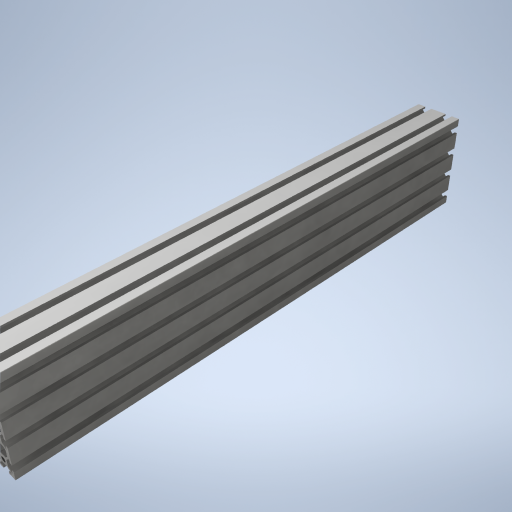
# Autodesk Inventor part: HFSP5-4080-425
Saved by Autodesk Inventor 2024 (Build 280153000, 153)
## iProperties
Category: PARTsolutions
Company: MISUMI
Created: 2024-08-01
Part Number: HFSP5-4080-425
Material: Aluminum 6061
Catalog Web Link: www.cadenas.de
Description: HFSP5-2040, HFSP5-2550, HFSP5-2060, HFSP5-2080, HFSP5-4060, HFSP5-4080-HFS5 Series -Aluminum Extrusion with Milled Surfaces/Rectangle (Vertical)-
Vendor: MISUMI
Document SubType Name: Modeling
Designer: psAdmin
Manufacturer: MISUMI
Mass: 1120.02 g
Surface Area: 3756.67 cm^2
Volume: 414.823 cm^3
Density: 2.7 g/cm^3
Appearance: Anodized - Light Gray
PSOL_IDENT_0: {$CADENAS_DATA/23d-libs/misumi/metric/38_al_extrusions_blackets/5/hfsp5_2040.prj},334 {VTYP=3D},{NB=
PSOL_IDENT_1: HFSP5-4080-425},{LINA=HFSP5-4080-425},{NN=HFSP5-2040, HFSP5-2550, HFSP5-2060, HFSP5-2080, HFSP5-4060
PSOL_IDENT_2: , HFSP5-4080},{DATE=31.05.2023 08:06:28},{GEOMDATE=27.07.2021 03:20:00},{VERSION=},{LINEID=130},{WBV
PSOL_IDENT_3: AR=L,ALT1,ALT10,NH10,AV,BV,CV,DV,EV,ALT12,Z,NH12,XA,XB,XC,XD,XE},{WBNUMERIC=L,NH10,AV,BV,CV,DV,EV,NH
PSOL_IDENT_4: 12,XA,XB,XC,XD,XE}  {NB=HFSP5-4080-425},{LINA=HFSP5-4080-425},{KT=DUMMY},{PN=HFSP5-4080-425},{TPS=HF
PSOL_IDENT_5: SP5-4080},{MAT=A6N01SS-T5  Aluminum Alloy},{ST=Anodize},{FRMH=80},{FRMW=40},{FRD=4.2},{L=425.0},{FS=
PSOL_IDENT_6: HFS5},{T=79.2},{A=40},{ALT1=},{M1=0},{IDM1=4.134},{DALT1=4.2},{DPL1=0},{DPR1=0},{ALT1PN=},{ALT10=},{
PSOL_IDENT_7: ALT10ALG= '','w/o Location Specified Wrench Access Hole Alteratons (Vertical)','1','with Location Sp
PSOL_IDENT_8: ecified Wrench Access Hole Alteratons (Vertical)' },{D6=N/A},{DD6=0},{DD6ALG=0},{DD6PN=},{NH10=0},{N
PSOL_IDENT_9: H10MAX=5},{NH10ALG=[0]},{AV=0.0},{AVMIN=7},{AVMAX=420},{AVALG=[0]},{BV=0.0},{BVMIN=2},{BVMAX=422},{B
PSOL_IDENT_10: VALG=[0]},{CV=0.0},{CVMIN=2},{CVMAX=424},{CVALG=[0]},{DV=0.0},{DVMIN=2},{DVMAX=426},{DVALG=[0]},{EV=
PSOL_IDENT_11: 0.0},{EVMIN=2},{EVMAX=418},{EVALG=[0]},{ALT9PN=},{ALT10PN=},{ALT11PN=},{ALT12=},{ALT12ALG= '','N/A'
PSOL_IDENT_12: },{Z=},{ZALG= '','N/A' },{DD12=0.0},{DD112=0.0},{NH12=0},{NH12MAX=5},{NH12ALG=[0]},{XA=0.0},{XAMIN=7
PSOL_IDENT_13: },{XAMAX=420},{XAALG=[0]},{XB=0.0},{XBMIN=2},{XBMAX=422},{XBALG=[0]},{XC=0.0},{XCMIN=2},{XCMAX=424},
PSOL_IDENT_14: {XCALG=[0]},{XD=0.0},{XDMIN=2},{XDMAX=426},{XDALG=[0]},{XE=0.0},{XEMIN=2},{XEMAX=418},{XEALG=[0]},{A
PSOL_IDENT_15: LT12PN=},{ERRORALT01=OK},{ERRORALT1012=OK},{ERRORPN=}
NB: HFSP5-4080-425
NN: HFSP5-2040, HFSP5-2550, HFSP5-2060, HFSP5-2080, HFSP5-4060, HFSP5-4080
NT: HFS5 Series -Aluminum Extrusion with Milled Surfaces/Rectangle (Vertical)-
NBSYN: $PN.
LINA: HFSP5-4080-425
CATALOG: Misumi
PN: HFSP5-4080-425
TPS: HFSP5-4080
MAT: A6N01SS-T5  Aluminum Alloy
ST: Clear Anodizing
L: 425
FS: HFS5
T: 79.2
A: 40
ALT1: w/o End Tapping
M1: 0
DPL1: 0
DPR1: 0
ALT10: w/o Location Specified Wrench Access Hole Alteratons (Vertical)
D6: N/A
NH10: 0
AV: 0
BV: 0
CV: 0
DV: 0
EV: 0
ALT12: N/A
Z: N/A
DD12: 0
DD112: 0
NH12: 0
XA: 0
XB: 0
XC: 0
XD: 0
XE: 0
SUPPLIER: MISUMI
ARTICLENO: HFSP5-4080-425
BOMINFO: HFSP5-4080-425
CREATOR: CADENAS GmbH
Title: HFSP5-4080-425
Author: Cadenas PARTsolutions
Comments: HFS5 Series -Aluminum Extrusion with Milled Surfaces/Rectangle (Vertical)-
Autodesk Inventor part; units mm, degrees
ref_plane "YZ Plane" through (0, 0, 0) normal (1, 0, 0) x (0, 1, 0)
ref_plane "XZ Plane" through (0, 0, 0) normal (0, 1, 0) x (-1, 0, 0)
ref_plane "XY Plane" through (0, 0, 0) normal (0, 0, 1) x (1, 0, 0)
sketch "Sketch_118" plane through (0, 0, 0) normal (0, 0, 1) x (1, 0, 0)
  line L0 (-20, -27) -> (-18, -27)
  line L1 (-18, -27) -> (-18, -24)
  line L2 (-18, -24) -> (-17.0607, -24)
  line L3 (-17.0607, -24) -> (-14, -27.0607)
  line L4 (-14, -27.0607) -> (-14, -29.4804)
  line L5 (-14, -29.4804) -> (-13.7, -30)
  line L6 (-13.7, -30) -> (-14, -30.5196)
  line L7 (-14, -30.5196) -> (-14, -32.9393)
  line L8 (-14, -32.9393) -> (-17.0607, -36)
  line L9 (-17.0607, -36) -> (-18, -36)
  line L10 (-18, -36) -> (-18, -33)
  line L11 (-18, -33) -> (-20, -33)
  line L12 (-20, -33) -> (-20, -39)
  arc A0 (-20, -39) -> (-19.8, -39.6) centre (-19, -39) ccw
  line L13 (-19.8, -39.6) -> (-13, -39.6)
  line L14 (-13, -39.6) -> (-13, -38)
  line L15 (-13, -38) -> (-16, -38)
  line L16 (-16, -38) -> (-16, -37.0607)
  line L17 (-16, -37.0607) -> (-12.9393, -34)
  line L18 (-12.9393, -34) -> (-10.5196, -34)
  line L19 (-10.5196, -34) -> (-10, -33.7)
  line L20 (-10, -33.7) -> (-9.4804, -34)
  line L21 (-9.4804, -34) -> (-7.0607, -34)
  line L22 (-7.0607, -34) -> (-4, -37.0607)
  line L23 (-4, -37.0607) -> (-4, -38)
  line L24 (-4, -38) -> (-7, -38)
  line L25 (-7, -38) -> (-7, -39.6)
  line L26 (-7, -39.6) -> (7, -39.6)
  line L27 (7, -39.6) -> (7, -38)
  line L28 (7, -38) -> (4, -38)
  line L29 (4, -38) -> (4, -37.0607)
  line L30 (4, -37.0607) -> (7.0607, -34)
  line L31 (7.0607, -34) -> (9.4804, -34)
  line L32 (9.4804, -34) -> (10, -33.7)
  line L33 (10, -33.7) -> (10.5196, -34)
  line L34 (10.5196, -34) -> (12.9393, -34)
  line L35 (12.9393, -34) -> (16, -37.0607)
  line L36 (16, -37.0607) -> (16, -38)
  line L37 (16, -38) -> (13, -38)
  line L38 (13, -38) -> (13, -39.6)
  line L39 (13, -39.6) -> (19.8, -39.6)
  arc A1 (19.8, -39.6) -> (20, -39) centre (19, -39) ccw
  line L40 (20, -39) -> (20, -33)
  line L41 (20, -33) -> (18, -33)
  line L42 (18, -33) -> (18, -36)
  line L43 (18, -36) -> (17.0607, -36)
  line L44 (17.0607, -36) -> (14, -32.9393)
  line L45 (14, -32.9393) -> (14, -30.5196)
  line L46 (14, -30.5196) -> (13.7, -30)
  line L47 (13.7, -30) -> (14, -29.4804)
  line L48 (14, -29.4804) -> (14, -27.0607)
  line L49 (14, -27.0607) -> (17.0607, -24)
  line L50 (17.0607, -24) -> (18, -24)
  line L51 (18, -24) -> (18, -27)
  line L52 (18, -27) -> (20, -27)
  line L53 (20, -27) -> (20, -13)
  line L54 (20, -13) -> (18, -13)
  line L55 (18, -13) -> (18, -16)
  line L56 (18, -16) -> (17.0607, -16)
  line L57 (17.0607, -16) -> (14, -12.9393)
  line L58 (14, -12.9393) -> (14, -10.5196)
  line L59 (14, -10.5196) -> (13.7, -10)
  line L60 (13.7, -10) -> (14, -9.4804)
  line L61 (14, -9.4804) -> (14, -7.0607)
  line L62 (14, -7.0607) -> (17.0607, -4)
  line L63 (17.0607, -4) -> (18, -4)
  line L64 (18, -4) -> (18, -7)
  line L65 (18, -7) -> (20, -7)
  line L66 (20, -7) -> (20, 7)
  line L67 (20, 7) -> (18, 7)
  line L68 (18, 7) -> (18, 4)
  line L69 (18, 4) -> (17.0607, 4)
  line L70 (17.0607, 4) -> (14, 7.0607)
  line L71 (14, 7.0607) -> (14, 9.4804)
  line L72 (14, 9.4804) -> (13.7, 10)
  line L73 (13.7, 10) -> (14, 10.5196)
  line L74 (14, 10.5196) -> (14, 12.9393)
  line L75 (14, 12.9393) -> (17.0607, 16)
  line L76 (17.0607, 16) -> (18, 16)
  line L77 (18, 16) -> (18, 13)
  line L78 (18, 13) -> (20, 13)
  line L79 (20, 13) -> (20, 27)
  line L80 (20, 27) -> (18, 27)
  line L81 (18, 27) -> (18, 24)
  line L82 (18, 24) -> (17.0607, 24)
  line L83 (17.0607, 24) -> (14, 27.0607)
  line L84 (14, 27.0607) -> (14, 29.4804)
  line L85 (14, 29.4804) -> (13.7, 30)
  line L86 (13.7, 30) -> (14, 30.5196)
  line L87 (14, 30.5196) -> (14, 32.9393)
  line L88 (14, 32.9393) -> (17.0607, 36)
  line L89 (17.0607, 36) -> (18, 36)
  line L90 (18, 36) -> (18, 33)
  line L91 (18, 33) -> (20, 33)
  line L92 (20, 33) -> (20, 39)
  arc A2 (20, 39) -> (19.8, 39.6) centre (19, 39) ccw
  line L93 (19.8, 39.6) -> (13, 39.6)
  line L94 (13, 39.6) -> (13, 38)
  line L95 (13, 38) -> (16, 38)
  line L96 (16, 38) -> (16, 37.0607)
  line L97 (16, 37.0607) -> (12.9393, 34)
  line L98 (12.9393, 34) -> (10.5196, 34)
  line L99 (10.5196, 34) -> (10, 33.7)
  line L100 (10, 33.7) -> (9.4804, 34)
  line L101 (9.4804, 34) -> (7.0607, 34)
  line L102 (7.0607, 34) -> (4, 37.0607)
  line L103 (4, 37.0607) -> (4, 38)
  line L104 (4, 38) -> (7, 38)
  line L105 (7, 38) -> (7, 39.6)
  line L106 (7, 39.6) -> (-7, 39.6)
  line L107 (-7, 39.6) -> (-7, 38)
  line L108 (-7, 38) -> (-4, 38)
  line L109 (-4, 38) -> (-4, 37.0607)
  line L110 (-4, 37.0607) -> (-7.0607, 34)
  line L111 (-7.0607, 34) -> (-9.4804, 34)
  line L112 (-9.4804, 34) -> (-10, 33.7)
  line L113 (-10, 33.7) -> (-10.5196, 34)
  line L114 (-10.5196, 34) -> (-12.9393, 34)
  line L115 (-12.9393, 34) -> (-16, 37.0607)
  line L116 (-16, 37.0607) -> (-16, 38)
  line L117 (-16, 38) -> (-13, 38)
  line L118 (-13, 38) -> (-13, 39.6)
  line L119 (-13, 39.6) -> (-19.8, 39.6)
  arc A3 (-19.8, 39.6) -> (-20, 39) centre (-19, 39) ccw
  line L120 (-20, 39) -> (-20, 33)
  line L121 (-20, 33) -> (-18, 33)
  line L122 (-18, 33) -> (-18, 36)
  line L123 (-18, 36) -> (-17.0607, 36)
  line L124 (-17.0607, 36) -> (-14, 32.9393)
  line L125 (-14, 32.9393) -> (-14, 30.5196)
  line L126 (-14, 30.5196) -> (-13.7, 30)
  line L127 (-13.7, 30) -> (-14, 29.4804)
  line L128 (-14, 29.4804) -> (-14, 27.0607)
  line L129 (-14, 27.0607) -> (-17.0607, 24)
  line L130 (-17.0607, 24) -> (-18, 24)
  line L131 (-18, 24) -> (-18, 27)
  line L132 (-18, 27) -> (-20, 27)
  line L133 (-20, 27) -> (-20, 13)
  line L134 (-20, 13) -> (-18, 13)
  line L135 (-18, 13) -> (-18, 16)
  line L136 (-18, 16) -> (-17.0607, 16)
  line L137 (-17.0607, 16) -> (-14, 12.9393)
  line L138 (-14, 12.9393) -> (-14, 10.5196)
  line L139 (-14, 10.5196) -> (-13.7, 10)
  line L140 (-13.7, 10) -> (-14, 9.4804)
  line L141 (-14, 9.4804) -> (-14, 7.0607)
  line L142 (-14, 7.0607) -> (-17.0607, 4)
  line L143 (-17.0607, 4) -> (-18, 4)
  line L144 (-18, 4) -> (-18, 7)
  line L145 (-18, 7) -> (-20, 7)
  line L146 (-20, 7) -> (-20, -7)
  line L147 (-20, -7) -> (-18, -7)
  line L148 (-18, -7) -> (-18, -4)
  line L149 (-18, -4) -> (-17.0607, -4)
  line L150 (-17.0607, -4) -> (-14, -7.0607)
  line L151 (-14, -7.0607) -> (-14, -9.4804)
  line L152 (-14, -9.4804) -> (-13.7, -10)
  line L153 (-13.7, -10) -> (-14, -10.5196)
  line L154 (-14, -10.5196) -> (-14, -12.9393)
  line L155 (-14, -12.9393) -> (-17.0607, -16)
  line L156 (-17.0607, -16) -> (-18, -16)
  line L157 (-18, -16) -> (-18, -13)
  line L158 (-18, -13) -> (-20, -13)
  line L159 (-20, -13) -> (-20, -27)
  line L160 (-16.5, 17.5607) -> (-14.4393, 15.5)
  line L161 (-14.4393, 15.5) -> (14.4393, 15.5)
  line L162 (14.4393, 15.5) -> (16.5, 17.5607)
  line L163 (16.5, 17.5607) -> (16.5, 22.4393)
  line L164 (16.5, 22.4393) -> (12.9393, 26)
  line L165 (12.9393, 26) -> (8, 26)
  arc A4 (6, 28) -> (8, 26) centre (8, 28) ccw
  line L166 (6, 28) -> (6, 32.9393)
  line L167 (6, 32.9393) -> (2.4393, 36.5)
  line L168 (2.4393, 36.5) -> (-2.4393, 36.5)
  line L169 (-2.4393, 36.5) -> (-6, 32.9393)
  line L170 (-6, 32.9393) -> (-6, 28)
  arc A5 (-8, 26) -> (-6, 28) centre (-8, 28) ccw
  line L171 (-8, 26) -> (-12.9393, 26)
  line L172 (-12.9393, 26) -> (-16.5, 22.4393)
  line L173 (-16.5, 22.4393) -> (-16.5, 17.5607)
  arc A6 (-16.5, -2.0251) -> (-16.2071, -2.7322) centre (-15.5, -2.0251) ccw
  line L174 (-16.2071, -2.7322) -> (-11.4489, -7.4905)
  line L175 (-11.4489, -7.4905) -> (-11.2757, -7.7904)
  arc A7 (-11.3801, -8.4172) -> (-11.2757, -7.7904) centre (-11.7087, -8.0404) ccw
  arc A8 (-11.3801, -8.4172) -> (-8.6199, -8.4172) centre (-10, -10) ccw
  arc A9 (-8.7243, -7.7904) -> (-8.6199, -8.4172) centre (-8.2913, -8.0404) ccw
  line L176 (-8.7243, -7.7904) -> (-7.8349, -6.25)
  arc A10 (-7.4019, -6) -> (-7.8349, -6.25) centre (-7.4019, -6.5) ccw
  line L177 (-7.4019, -6) -> (-6.5, -6)
  arc A11 (-6, -6.5) -> (-6.5, -6) centre (-6.5, -6.5) ccw
  line L178 (-6, -6.5) -> (-6, -13)
  arc A12 (-6, -13) -> (-5, -14) centre (-5, -13) ccw
  line L179 (-5, -14) -> (5, -14)
  arc A13 (5, -14) -> (6, -13) centre (5, -13) ccw
  line L180 (6, -13) -> (6, -6.5)
  arc A14 (6.5, -6) -> (6, -6.5) centre (6.5, -6.5) ccw
  line L181 (6.5, -6) -> (7.4019, -6)
  arc A15 (7.8349, -6.25) -> (7.4019, -6) centre (7.4019, -6.5) ccw
  line L182 (7.8349, -6.25) -> (8.7243, -7.7904)
  arc A16 (8.6199, -8.4172) -> (8.7243, -7.7904) centre (8.2913, -8.0404) ccw
  arc A17 (8.6199, -8.4172) -> (11.3801, -8.4172) centre (10, -10) ccw
  arc A18 (11.2757, -7.7904) -> (11.3801, -8.4172) centre (11.7087, -8.0404) ccw
  line L183 (11.2757, -7.7904) -> (11.4489, -7.4905)
  line L184 (11.4489, -7.4905) -> (16.2071, -2.7322)
  arc A19 (16.2071, -2.7322) -> (16.5, -2.0251) centre (15.5, -2.0251) ccw
  line L185 (16.5, -2.0251) -> (16.5, 2.0251)
  arc A20 (16.5, 2.0251) -> (16.2071, 2.7322) centre (15.5, 2.0251) ccw
  line L186 (16.2071, 2.7322) -> (11.4489, 7.4905)
  line L187 (11.4489, 7.4905) -> (11.2757, 7.7904)
  arc A21 (11.3801, 8.4172) -> (11.2757, 7.7904) centre (11.7087, 8.0404) ccw
  arc A22 (11.3801, 8.4172) -> (8.6199, 8.4172) centre (10, 10) ccw
  arc A23 (8.7243, 7.7904) -> (8.6199, 8.4172) centre (8.2913, 8.0404) ccw
  line L188 (8.7243, 7.7904) -> (7.8349, 6.25)
  arc A24 (7.4019, 6) -> (7.8349, 6.25) centre (7.4019, 6.5) ccw
  line L189 (7.4019, 6) -> (6.5, 6)
  arc A25 (6, 6.5) -> (6.5, 6) centre (6.5, 6.5) ccw
  line L190 (6, 6.5) -> (6, 13)
  arc A26 (6, 13) -> (5, 14) centre (5, 13) ccw
  line L191 (5, 14) -> (-5, 14)
  arc A27 (-5, 14) -> (-6, 13) centre (-5, 13) ccw
  line L192 (-6, 13) -> (-6, 6.5)
  arc A28 (-6.5, 6) -> (-6, 6.5) centre (-6.5, 6.5) ccw
  line L193 (-6.5, 6) -> (-7.4019, 6)
  arc A29 (-7.8349, 6.25) -> (-7.4019, 6) centre (-7.4019, 6.5) ccw
  line L194 (-7.8349, 6.25) -> (-8.7243, 7.7904)
  arc A30 (-8.6199, 8.4172) -> (-8.7243, 7.7904) centre (-8.2913, 8.0404) ccw
  arc A31 (-8.6199, 8.4172) -> (-11.3801, 8.4172) centre (-10, 10) ccw
  arc A32 (-11.2757, 7.7904) -> (-11.3801, 8.4172) centre (-11.7087, 8.0404) ccw
  line L195 (-11.2757, 7.7904) -> (-11.4489, 7.4905)
  line L196 (-11.4489, 7.4905) -> (-16.2071, 2.7322)
  arc A33 (-16.2071, 2.7322) -> (-16.5, 2.0251) centre (-15.5, 2.0251) ccw
  line L197 (-16.5, 2.0251) -> (-16.5, -2.0251)
  line L198 (-16.5, -17.5607) -> (-16.5, -22.4393)
  line L199 (-16.5, -22.4393) -> (-12.9393, -26)
  line L200 (-12.9393, -26) -> (-8, -26)
  arc A34 (-6, -28) -> (-8, -26) centre (-8, -28) ccw
  line L201 (-6, -28) -> (-6, -32.9393)
  line L202 (-6, -32.9393) -> (-2.4393, -36.5)
  line L203 (-2.4393, -36.5) -> (2.4393, -36.5)
  line L204 (2.4393, -36.5) -> (6, -32.9393)
  line L205 (6, -32.9393) -> (6, -28)
  arc A35 (8, -26) -> (6, -28) centre (8, -28) ccw
  line L206 (8, -26) -> (12.9393, -26)
  line L207 (12.9393, -26) -> (16.5, -22.4393)
  line L208 (16.5, -22.4393) -> (16.5, -17.5607)
  line L209 (16.5, -17.5607) -> (14.4393, -15.5)
  line L210 (14.4393, -15.5) -> (-14.4393, -15.5)
  line L211 (-14.4393, -15.5) -> (-16.5, -17.5607)
  constraints: 424 end point, 72 point on circle, 36 centre point
extrude "Extrusion1" add sketch "Sketch_118" against normal blind 425
sketch "Sketch2" plane through (0, 0, -425) normal (0, 0, -1) x (-1, 0, 0)
  point P0 (-10, 30)
hole "Hole1" at (10, 30, -425) direction (0, 0, 1) diameter 4.2 depth 425
pattern_linear "Rectangular Pattern1" count 2 spacing 20 along (-1, 0, 0) count 2 spacing 60 along (0, -1, 0) of "Hole1"
thread "Thread2" size "M4.5x0.75" class "6H" standard "ANSI Metric M Profile" length 10
thread "Thread3" size "M5x0.8" class "6H" standard "ANSI Metric M Profile" length 10
thread "Thread4" size "M5x0.8" class "6H" standard "ANSI Metric M Profile" length 10
thread "Thread5" size "M5x0.8" class "6H" standard "ANSI Metric M Profile" length 10
thread "Thread6" size "M5x0.8" class "6H" standard "ANSI Metric M Profile" length 10
thread "Thread7" size "M5x0.8" class "6H" standard "ANSI Metric M Profile" length 10
thread "Thread8" size "M5x0.8" class "6H" standard "ANSI Metric M Profile" length 10
thread "Thread9" size "M5x0.8" class "6H" standard "ANSI Metric M Profile" length 10
thread "Thread10" size "M5x0.8" class "6H" standard "ANSI Metric M Profile" length 10
thread "Thread11" size "M5x0.8" class "6H" standard "ANSI Metric M Profile" length 10
thread "Thread12" size "M5x0.8" class "6H" standard "ANSI Metric M Profile" length 10
thread "Thread13" size "M5x0.8" class "6H" standard "ANSI Metric M Profile" length 10
thread "Thread14" size "M5x0.8" class "6H" standard "ANSI Metric M Profile" length 10
thread "Thread15" size "M5x0.8" class "6H" standard "ANSI Metric M Profile" length 10
thread "Thread16" size "M5x0.8" class "6H" standard "ANSI Metric M Profile" length 10
thread "Thread17" size "M5x0.8" class "6H" standard "ANSI Metric M Profile" length 10
body "Solid1"
